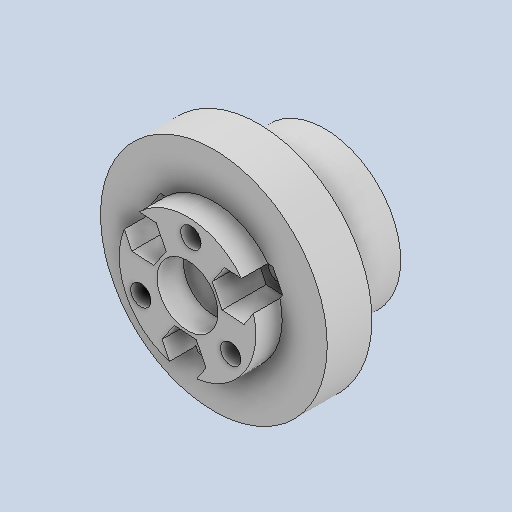
# Autodesk Inventor part: Os
Saved by Autodesk Inventor 2022 (Build 260153000, 153)
## iProperties
Created: 2023-01-20
Part Number: Os
Material: Generic
Document SubType Name: Modeling
Designer: Kamil
Density: 1 g/cm^3
Appearance: Default
Author: Kamil
Autodesk Inventor part; units mm, degrees
ref_plane "YZ Plane" through (0, 0, 0) normal (1, 0, 0) x (0, 1, 0)
ref_plane "XZ Plane" through (0, 0, 0) normal (0, 1, 0) x (-1, 0, 0)
ref_plane "XY Plane" through (0, 0, 0) normal (0, 0, 1) x (1, 0, 0)
sketch "Sketch1" plane through (0, 0, 0) normal (0, 0, 1) x (1, 0, 0)
  circle A0 centre (0, 0) radius 23.3333 projected
  arc A1 (-39.2843, 4.1223) -> (-36.4252, -2.8784) centre (-31.328, 3.2874) ccw projected
  arc A2 (-35.6202, -8.1415) -> (-36.4252, -2.8784) centre (-38.9739, -5.9614) ccw projected
  arc A3 (-35.6202, -8.1415) -> (-36.2558, -15.6768) centre (-28.9129, -12.5018) ccw projected
  arc A4 (-36.2558, -15.6768) -> (33.8969, -20.2792) centre (0, 0) ccw projected
  arc A5 (33.8969, -20.2792) -> (34.2512, -12.7254) centre (27.0317, -16.172) ccw projected
  arc A6 (35.737, -7.6127) -> (34.2512, -12.7254) centre (37.861, -11.0021) ccw projected
  arc A7 (35.737, -7.6127) -> (39.4862, -1.0454) centre (31.489, -0.8337) ccw projected
  arc A8 (39.4862, -1.0454) -> (-39.2843, 4.1223) centre (0, 0) ccw projected
  circle A9 centre (-9.1932, -4.5329) radius 2 projected
  circle A10 centre (9.1932, 4.5329) radius 2 projected
  circle A11 centre (-0.671, -10.228) radius 2 projected
  circle A12 centre (-8.5222, 5.6951) radius 2 projected
  circle A13 centre (0.671, 10.228) radius 2 projected
  circle A14 centre (8.5222, -5.6951) radius 2 projected
  circle A15 centre (0, 0) radius 13.4591 projected
  line L0 (-5.9382, 0.859) -> (-7.1311, 0.7284) projected
  arc A16 (-5.6118, -2.1232) -> (-5.9382, 0.859) centre (0, 0) ccw projected
  line L1 (-6.8047, -2.2538) -> (-5.6118, -2.1232) projected
  line L2 (-7.1311, 0.7284) -> (-6.8047, -2.2538) projected
  line L3 (23.3333, 0) -> (22.3333, 0)
  circle A17 centre (0, 0) radius 22.3333
  circle A18 centre (0, 0) radius 6
  circle A19 centre (16.7628, -26.571) radius 3.75 projected
  circle A20 centre (-29.1794, 11.6435) radius 3.75 projected
  circle A21 centre (2.0567, 31.3493) radius 3.75 projected
  circle A22 centre (-20.0905, -24.1532) radius 3.75 projected
  circle A23 centre (30.4505, 7.7314) radius 3.75 projected
  point P0 (0, 0)
  dimension "d0" = 1
  constraints: 2 coincident, 2 end point, 2 horizontal alignment, 1 horizontal, 6 other
  measures "d0" distance of L3.start L3.end
extrude "Extrusion1" add sketch "Sketch1" along normal blind 3.8 contours A15 | A18 L1 L2 L0 | A16 A18 | A17
sketch "Sketch2" plane through (0, 0, 0) normal (0, 0, -1) x (-1, 0, 0)
  circle A0 centre (0, 0) radius 15 projected
  circle A1 centre (0, 0) radius 22.3333 projected
  circle A2 centre (9.1932, -4.5329) radius 2 projected
  circle A3 centre (-9.1932, 4.5329) radius 2 projected
  circle A4 centre (0.671, -10.228) radius 2 projected
  circle A5 centre (8.5222, 5.6951) radius 2 projected
  circle A6 centre (-0.671, 10.228) radius 2 projected
  circle A7 centre (-8.5222, -5.6951) radius 2 projected
  point P0 (0, 0)
ref_plane "Work Plane1" through (-21.6708, -21.6708, -13) normal (0, 0, -1) x (0, 1, 0)
extrude "Extrusion2" add sketch "Sketch2" along normal up to surface (13 mm away) contours A0
sketch "Sketch3" plane through (0, 0, 3.8) normal (0, 0, 1) x (1, 0, 0)
  point P0 (0, 0)
sketch "Sketch4" plane through (0, 0, -13) normal (0, 0, -1) x (-1, 0, 0)
  circle A0 centre (0, 0) radius 15 projected
  circle A1 centre (-8.5222, -5.6951) radius 2 projected
  circle A2 centre (-0.671, 10.228) radius 2 projected
  circle A3 centre (8.5222, 5.6951) radius 2 projected
  circle A4 centre (0.671, -10.228) radius 2 projected
  circle A5 centre (-9.1932, 4.5329) radius 2 projected
  circle A6 centre (9.1932, -4.5329) radius 2 projected
  line L0 (0, 0) -> (9.1932, -4.5329)
  line L1 (9.1932, -4.5329) -> (12.3324, -6.0807)
  circle A7 centre (9.1932, -4.5329) radius 2 projected
  circle A8 centre (9.1932, -4.5329) radius 3.5
  circle A9 centre (8.5222, 5.6951) radius 3.5
  circle A10 centre (-0.671, 10.228) radius 3.5
  circle A11 centre (-9.1932, 4.5329) radius 3.5
  circle A12 centre (-8.5222, -5.6951) radius 3.5
  circle A13 centre (0.671, -10.228) radius 3.5
  point P0 (0, 0)
  point P1 (11.4322, 7.6398)
  point P2 (-0.9001, 13.7205)
  point P3 (-12.3324, 6.0807)
  point P4 (-11.4322, -7.6398)
  point P5 (0.9001, -13.7205)
  dimension "d5" = 3.5
  dimension "d8" = 360
  constraints: 4 end point, 1 coincident, 1 collinear, 37 other
  measures "d5" distance of L0.end L1.end
extrude "Extrusion3" cut sketch "Sketch4" against normal blind 5 contours A1 | A6 L1 L0 | A6 L0 A8 L1 | L0 L1 A6 | A6 L1 A8 L0 | A10 | A12
sketch "Sketch5" plane through (0, 0, 3.8) normal (0, 0, 1) x (1, 0, 0)
  circle A0 centre (0, 0) radius 22.3333 projected
  circle A1 centre (-9.1932, -4.5329) radius 2 projected
  circle A2 centre (9.1932, 4.5329) radius 2 projected
  circle A3 centre (-0.671, -10.228) radius 2 projected
  circle A4 centre (-8.5222, 5.6951) radius 2 projected
  circle A5 centre (0.671, 10.228) radius 2 projected
  circle A6 centre (8.5222, -5.6951) radius 2 projected
  line L0 (0, 0) -> (-0.671, -10.228)
  circle A7 centre (-0.671, -10.228) radius 2 projected
  line L1 (-0.671, -10.228) -> (-1.462, -22.2854)
  circle A8 centre (0, 0) radius 22.3333 projected
  line L2 (-0.671, -10.228) -> (-0.9001, -13.7205)
  line L3 (-3.0871, -13.8731) -> (-5.0083, -9.9765)
  line L4 (-5.0083, -9.9765) -> (-2.5944, -6.3644)
  line L5 (-2.5944, -6.3644) -> (1.7407, -6.6488)
  line L6 (1.7407, -6.6488) -> (3.662, -10.5454)
  line L7 (3.662, -10.5454) -> (1.2481, -14.1575)
  line L8 (1.2481, -14.1575) -> (-3.0871, -13.8731)
  line L9 (4.2145, -5.429) -> (6.6284, -1.8169)
  line L10 (6.1358, -9.3256) -> (4.2145, -5.429)
  line L11 (10.4709, -9.61) -> (6.1358, -9.3256)
  line L12 (12.8848, -5.9979) -> (10.4709, -9.61)
  line L13 (10.9635, -2.1013) -> (12.8848, -5.9979)
  line L14 (6.6284, -1.8169) -> (10.9635, -2.1013)
  line L15 (6.8089, 0.9353) -> (4.8877, 4.8319)
  line L16 (11.1441, 0.6509) -> (6.8089, 0.9353)
  line L17 (13.558, 4.2631) -> (11.1441, 0.6509)
  line L18 (11.6367, 8.1596) -> (13.558, 4.2631)
  line L19 (7.3016, 8.4441) -> (11.6367, 8.1596)
  line L20 (4.8877, 4.8319) -> (7.3016, 8.4441)
  line L21 (2.5944, 6.3644) -> (-1.7407, 6.6488)
  line L22 (5.0083, 9.9765) -> (2.5944, 6.3644)
  line L23 (3.0871, 13.8731) -> (5.0083, 9.9765)
  line L24 (-1.2481, 14.1575) -> (3.0871, 13.8731)
  line L25 (-3.662, 10.5454) -> (-1.2481, 14.1575)
  line L26 (-1.7407, 6.6488) -> (-3.662, 10.5454)
  line L27 (-4.2145, 5.429) -> (-6.6284, 1.8169)
  line L28 (-6.1358, 9.3256) -> (-4.2145, 5.429)
  line L29 (-10.4709, 9.61) -> (-6.1358, 9.3256)
  line L30 (-12.8848, 5.9979) -> (-10.4709, 9.61)
  line L31 (-10.9635, 2.1013) -> (-12.8848, 5.9979)
  line L32 (-6.6284, 1.8169) -> (-10.9635, 2.1013)
  line L33 (-6.8089, -0.9353) -> (-4.8877, -4.8319)
  line L34 (-11.1441, -0.6509) -> (-6.8089, -0.9353)
  line L35 (-13.558, -4.2631) -> (-11.1441, -0.6509)
  line L36 (-11.6367, -8.1596) -> (-13.558, -4.2631)
  line L37 (-7.3016, -8.4441) -> (-11.6367, -8.1596)
  line L38 (-4.8877, -4.8319) -> (-7.3016, -8.4441)
  point P0 (0, 0)
  point P1 (-0.6732, -10.261)
  point P2 (-0.9195, -14.0153)
  point P3 (11.6779, -7.8039)
  point P4 (12.5974, 6.2114)
  point P5 (0.9195, 14.0153)
  point P6 (-11.6779, 7.8039)
  point P7 (-12.5974, -6.2114)
  dimension "d13" = 3.5
  dimension "d16" = 360
  constraints: 78 end point, 2 point on line, 1 collinear, 1 midpoint, 94 other
  measures "d13" distance of L1.start L2.end
extrude "Extrusion4" add sketch "Sketch5" along normal blind 5 contours A0 | L9 L14 L13 L12 L11 L10 | L21 L26 L25 L24 L23 L22 | L33 L38 L37 L36 L35 L34
sketch "Sketch6" plane through (0, 0, 3.8) normal (0, 0, 1) x (1, 0, 0)
  line L0 (6.8089, 0.9353) -> (11.1441, 0.6509) projected
  line L1 (11.1441, 0.6509) -> (13.558, 4.2631) projected
  line L2 (13.558, 4.2631) -> (11.6367, 8.1596) projected
  line L3 (11.6367, 8.1596) -> (7.3016, 8.4441) projected
  line L4 (7.3016, 8.4441) -> (4.8877, 4.8319) projected
  line L5 (4.8877, 4.8319) -> (6.8089, 0.9353) projected
  circle A0 centre (9.1932, 4.5329) radius 2 projected
  circle A1 centre (0, 0) radius 22.3333 projected
  circle A2 centre (8.5222, -5.6951) radius 2 projected
  circle A3 centre (0.671, 10.228) radius 2 projected
  circle A4 centre (-9.1932, -4.5329) radius 2 projected
  line L6 (1.2481, -14.1575) -> (-3.0871, -13.8731) projected
  line L7 (-3.0871, -13.8731) -> (-5.0083, -9.9765) projected
  line L8 (-5.0083, -9.9765) -> (-2.5944, -6.3644) projected
  line L9 (-2.5944, -6.3644) -> (1.7407, -6.6488) projected
  line L10 (1.7407, -6.6488) -> (3.662, -10.5454) projected
  line L11 (3.662, -10.5454) -> (1.2481, -14.1575) projected
  line L12 (-4.2145, 5.429) -> (-6.6284, 1.8169) projected
  line L13 (-6.6284, 1.8169) -> (-10.9635, 2.1013) projected
  line L14 (-10.9635, 2.1013) -> (-12.8848, 5.9979) projected
  line L15 (-12.8848, 5.9979) -> (-10.4709, 9.61) projected
  line L16 (-10.4709, 9.61) -> (-6.1358, 9.3256) projected
  line L17 (-6.1358, 9.3256) -> (-4.2145, 5.429) projected
  line L18 (6.8089, 0.9353) -> (4.8877, 4.8319) projected
  line L19 (4.8877, 4.8319) -> (7.3016, 8.4441) projected
  line L20 (7.3016, 8.4441) -> (11.6367, 8.1596) projected
  line L21 (11.6367, 8.1596) -> (13.558, 4.2631) projected
  line L22 (13.558, 4.2631) -> (11.1441, 0.6509) projected
  line L23 (11.1441, 0.6509) -> (6.8089, 0.9353) projected
  circle A5 centre (-0.671, -10.228) radius 2 projected
  circle A6 centre (-8.5222, 5.6951) radius 2 projected
  point P0 (0, 0)
extrude "Extrusion5" add sketch "Sketch6" along normal blind 1.5 contours L5 L4 L3 L2 L1 L0 | L6 L7 L8 L9 L10 L11 | L12 L13 L14 L15 L16 L17
sketch "Sketch7" plane through (0, 0, 8.8) normal (0, 0, 1) x (1, 0, 0)
  circle A0 centre (8.5222, -5.6951) radius 2 projected
  circle A1 centre (9.1932, 4.5329) radius 2 projected
  circle A2 centre (-0.671, -10.228) radius 2 projected
  circle A3 centre (0.671, 10.228) radius 2 projected
  circle A4 centre (-9.1932, -4.5329) radius 2 projected
  arc A5 (5.9995, 0.0758) -> (5.2863, -2.8382) centre (0, 0) ccw projected
  line L0 (7.1651, -0.2095) -> (5.9995, 0.0758) projected
  line L1 (6.4519, -3.1235) -> (7.1651, -0.2095) projected
  line L2 (5.2863, -2.8382) -> (6.4519, -3.1235) projected
  circle A6 centre (-8.5222, 5.6951) radius 2 projected
  circle A7 centre (0, 0) radius 13.4542 projected
  circle A8 centre (0, 0) radius 6
  circle A9 centre (0, 0) radius 22.3333 projected
  circle A10 centre (8.5222, -5.6951) radius 2 projected
  circle A11 centre (0.671, 10.228) radius 2 projected
  circle A12 centre (-9.1932, -4.5329) radius 2 projected
  line L3 (1.2481, -14.1575) -> (-3.0871, -13.8731) projected
  line L4 (-3.0871, -13.8731) -> (-5.0083, -9.9765) projected
  line L5 (-5.0083, -9.9765) -> (-2.5944, -6.3644) projected
  line L6 (-2.5944, -6.3644) -> (1.7407, -6.6488) projected
  line L7 (1.7407, -6.6488) -> (3.662, -10.5454) projected
  line L8 (3.662, -10.5454) -> (1.2481, -14.1575) projected
  line L9 (-4.2145, 5.429) -> (-6.6284, 1.8169) projected
  line L10 (-6.6284, 1.8169) -> (-10.9635, 2.1013) projected
  line L11 (-10.9635, 2.1013) -> (-12.8848, 5.9979) projected
  line L12 (-12.8848, 5.9979) -> (-10.4709, 9.61) projected
  line L13 (-10.4709, 9.61) -> (-6.1358, 9.3256) projected
  line L14 (-6.1358, 9.3256) -> (-4.2145, 5.429) projected
  line L15 (6.8089, 0.9353) -> (4.8877, 4.8319) projected
  line L16 (4.8877, 4.8319) -> (7.3016, 8.4441) projected
  line L17 (7.3016, 8.4441) -> (11.6367, 8.1596) projected
  line L18 (11.6367, 8.1596) -> (13.558, 4.2631) projected
  line L19 (13.558, 4.2631) -> (11.1441, 0.6509) projected
  line L20 (11.1441, 0.6509) -> (6.8089, 0.9353) projected
  point P0 (0, 0)
  point P1 (1.7989, -13.3334)
  point P2 (13.0072, 3.4389)
  point P3 (10.6476, 8.2245)
  point P4 (-9.4818, 9.5451)
  point P5 (-12.4465, 5.1088)
  point P6 (-3.5254, -12.9841)
  point P7 (5.9995, 0.0758)
  constraints: 1 coincident, 3 other
extrude "Extrusion6" add sketch "Sketch7" along normal blind 5.2 contours L0 L1 L2 A8 | A7 L8 L7 L6 L5 L4 L11 L10 L9 L14 L13 L17 L16 L15 L20 L19
body "Solid1"
